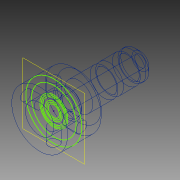
# Autodesk Inventor part: Extender
Saved by Autodesk Inventor 2015 (Build 190159000, 159)
## iProperties
Created: 2015-01-06
Part Number: Extender
Material: Aluminum 6061
Document SubType Name: Modeling
Designer: ice
Mass: 1.90852 g
Surface Area: 13.1319 cm^2
Volume: 1.90852 cm^3
Density: 2.7 g/cm^3
Appearance: Aluminum - Flat
Author: ice
Autodesk Inventor part; units mm, degrees
sketch "Sketch1" plane through (0, 0, 0) normal (1, 0, 0) x (0, 1, 0)
  line L0 (0, 0) -> (31.6248, 0)
  line L1 (30, 1) -> (30, 2.5)
  line L2 (27.5, 2.5) -> (24.5, 2.5)
  arc A0 (27.5, 2.5) -> (28.5, 2.5) centre (28, 2.5) ccw
  arc A1 (23.5, 2.5) -> (24.5, 2.5) centre (24, 2.5) ccw
  line L3 (19, 5) -> (19, 2.5)
  line L4 (23.5, 2.5) -> (22, 2.5)
  line L5 (22, 2.5) -> (19, 2.5)
  line L6 (30, 2.5) -> (28.5, 2.5)
  line L7 (12, 5) -> (19, 5)
  line L8 (17, 1.25) -> (17, 1)
  arc A2 (17, 1.25) -> (17, 2.25) centre (17, 1.75) ccw
  line L9 (19, 5) -> (19, 4)
  line L10 (19, 5) -> (18, 5)
  line L11 (12, 5) -> (12, 2.55)
  line L12 (12, 2.55) -> (17, 2.55)
  line L13 (17, 2.55) -> (17, 2.25)
  line L14 (30, 2.5) -> (30, 0)
  line L15 (17, 1) -> (17, 0)
  line L16 (17, 0) -> (30, 0)
  dimension "d50" = 1.5
  dimension "d63" = 1
  dimension "d64" = 3
  dimension "d65" = 1
  dimension "d77" = 1
  dimension "d78" = 2.5
  dimension "d79" = 1.5
  dimension "d94" = 1.5
  dimension "d95" = 3
  dimension "d99" = 8
  dimension "d134" = 7
  dimension "d141" = 0.25
  dimension "d166" = 1
  dimension "d167" = 1
  dimension "d168" = 5
  dimension "d170" = 4.5
  dimension "d171" = 11
  dimension "d172" = 2.45
  dimension "d173" = 1.75
  dimension "d174" = 1
  dimension "d175" = 18
  constraints: 34 end point, 7 point on circle, 6 point on line, 4 vertical, 3 centre point, 3 horizontal, 2 collinear, 2 perpendicular
  measures "d50" distance of L1.end L6.end
  measures "d63" distance of L6.end L2.start
  measures "d64" distance of L2.end L2.start
  measures "d65" distance of A1.start L2.end
  measures "d77" distance from line of L0 L1.start
  measures "d78" distance from line of L0 L1.end
  measures "d79" distance of L1.start L1.end
  measures "d94" distance of L4.start L4.end
  measures "d95" distance of L4.end L3.end
  measures "d99" distance of L1.end L4.end
  measures "d134" distance of L7.start L3.start
  measures "d141" distance of L8.start L8.end
  measures "d166" distance of L3.start L9.end
  measures "d167" distance of L3.start L10.end
  measures "d168" distance from line of L0 L7.start
  measures "d170" distance of L3.end A1.start
  measures "d171" distance of L3.end L1.end
  measures "d172" distance of L7.start L11.end
  measures "d173" distance from line of L0 A2.centre
  measures "d174" distance of L8.start L13.end
  measures "d175" horizontal distance of L7.start L1.end
revolve "Revolution1" add sketch "Sketch1" angle 360 about axis through (0, 0, 0) along (0, 1, 0)
ref_plane "Work Plane2" through (0, 0, 5) normal (0, 0, 1) x (1, 0, 0)
sketch "Sketch5" plane through (0, 0, 5) normal (0, 0, 1) x (1, 0, 0)
  line L0 (5, -4) -> (-5, -4) projected
  line L1 (5, 12) -> (-5, 12) projected
  circle A0 centre (0, 14.5) radius 0.95
  dimension "d144" = 1.9
  constraints: 1 centre point
  measures "d144" diameter of A0
hole "Hole1" at (0, 14.5, 5) direction (0, 0, -1) diameter 1.9 end through all
chamfer "Chamfer3" distance 1 angle 45 1 edges at (0, 30, -2.5)
ref_plane "Work Plane3" through (5, 0, 0) normal (1, 0, 0) x (0, 1, 0)
sketch "Sketch6" plane through (5, 0, 0) normal (1, 0, 0) x (0, 1, 0)
  line L0 (12, -5) -> (12, 5) projected
  circle A0 centre (14.5, 0) radius 0.95
  point P0 (0, 0)
  dimension "d147" = 1.9
  constraints: 1 centre point
  measures "d147" diameter of A0
hole "Hole2" at (5, 14.5, 0) direction (-1, 0, 0) diameter 1.9 end through all
thread "Thread5" size "M2x0.4" class "6H" standard "ANSI Metric M Profile" full length
thread "Thread6" size "M2x0.4" class "6H" standard "ANSI Metric M Profile" full length
thread "Thread7" size "M2x0.4" class "6H" standard "ANSI Metric M Profile" full length
thread "Thread8" size "M2x0.4" class "6H" standard "ANSI Metric M Profile" full length
chamfer "Chamfer4" distance 1 angle 45 1 edges at (0, 19, -5)
sketch "Sketch7" plane through (0, 30, 0) normal (0, 1, 0) x (1, 0, 0)
  circle A0 centre (0, 0) radius 1
  dimension "d176" = 2
  constraints: 1 centre point, 1 coincident
  measures "d176" diameter of A0
hole "Hole3" at (0, 30, 0) direction (0, -1, 0) diameter 2 end through all
ref_plane "Work Plane4" through (0, 14.5, 0) normal (0, 1, 0) x (-1, 0, 0)
sketch "Sketch8" plane through (0, 14.5, 0) normal (0, 1, 0) x (-1, 0, 0)
  circle A0 centre (0, 0) radius 5
  circle A1 centre (0, 0) radius 4
  circle A2 centre (0, 0) radius 1.25 projected
  circle A3 centre (0, 0) radius 2.5
  circle A4 centre (0, 0) radius 2.25
  circle A5 centre (0, 0) radius 1.25
  circle A6 centre (0, 0) radius 1
  circle A7 centre (0, 0) radius 1.5
  circle A8 centre (0, 0) radius 2
  constraints: 8 centre point, 8 coincident
body "Solid1"
